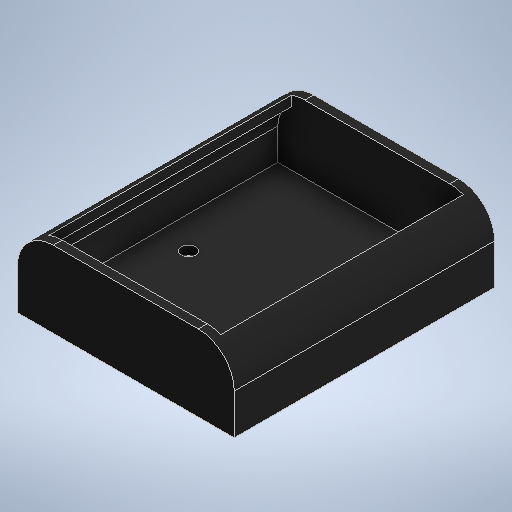
# Autodesk Inventor part: battery_box
Saved by Autodesk Inventor 2026.1 (Build 301233020, 233B)
## iProperties
Created: 2026-01-22
Part Number: battery_box
Material: 一般
Document SubType Name: Modeling
Designer: hibik
Density: 1 g/cm^3
Appearance: 既定
Author: hibik
Autodesk Inventor part; units mm, degrees
ref_plane "YZ Plane" through (0, 0, 0) normal (1, 0, 0) x (0, 1, 0)
ref_plane "XZ Plane" through (0, 0, 0) normal (0, 1, 0) x (-1, 0, 0)
ref_plane "XY Plane" through (0, 0, 0) normal (0, 0, 1) x (1, 0, 0)
sketch "スケッチ1" plane through (0, 0, 0) normal (0, 1, 0) x (-1, 0, 0)
  line L0 (-24.15, -29) -> (24.15, -29)
  line L1 (24.15, -29) -> (24.15, 29)
  line L2 (24.15, 29) -> (-24.15, 29)
  line L3 (-24.15, 29) -> (-24.15, -29)
  line L4 (-24.15, -29) -> (24.15, 29) construction
  line L5 (24.15, -29) -> (-24.15, 29) construction
  point P0 (0, 0)
  dimension "d0" = 48.3
  dimension "d1" = 58
  constraints: 12 end point, 2 midpoint, 2 parallel, 1 horizontal, 1 perpendicular
  measures "d0" distance of L2.end L1.end
  measures "d1" distance of L1.end L0.end
extrude "押し出し1" add sketch "スケッチ1" along normal blind 17
fillet "フィレット1" radius 8 2 edges at (24.15, 17, 0) (-24.15, 17, 0)
shell "シェル1" thickness 2 removed faces 0
sketch "スケッチ2" plane through (0, 17, 0) normal (0, 1, 0) x (1, 0, 0)
  line L0 (22.15, 27) -> (-22.15, 27) projected
  line L1 (19.15, -27) -> (-19.15, -27)
  line L2 (-19.15, -27) -> (-19.15, 27)
  line L3 (-19.15, 27) -> (19.15, 27)
  line L4 (19.15, 27) -> (19.15, -27)
  line L5 (19.15, -27) -> (-19.15, 27) construction
  line L6 (-19.15, -27) -> (19.15, 27) construction
  line L7 (-16.15, -29) -> (-16.15, 29) projected
  point P0 (0, 0)
  dimension "d8" = 3
  constraints: 12 end point, 2 midpoint, 2 parallel, 1 horizontal, 1 perpendicular, 1 point on line
  measures "d8" distance between parallel lines of L7 L2
extrude "押し出し2" cut sketch "スケッチ2" against normal blind 5
sketch "スケッチ3" plane through (-22.15, 2, 27) normal (0, 1, 0) x (1, 0, 0)
  circle A0 centre (37.15, 27) radius 1.6
  circle A1 centre (7.15, 27) radius 1.6
  line L0 (6, 54) -> (38.3, 54) projected
  line L1 (22.15, 54) -> (22.15, 0) construction
  line L2 (0, 0) -> (44.3, 0) projected
  point P0 (22.15, 27)
  dimension "d9" = 3.2
  dimension "d11" = 30
  constraints: 2 centre point, 2 end point, 2 midpoint, 1 horizontal alignment, 1 other
  measures "d9" diameter of A0
  measures "d11" distance of A0.centre A1.centre
extrude "押し出し3" cut sketch "スケッチ3" against normal through all
